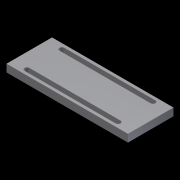
# Autodesk Inventor part: JointA3
Saved by Autodesk Inventor 2011 (Build 150239000, 239)
## iProperties
Created: 2012-10-15
Part Number: JointA3
Document SubType Name: Modeling
Designer: JohnHenry
Density: 1 g/cm^3
Author: JohnHenry
Autodesk Inventor part; units mm, degrees
ref_plane "YZ Plane" through (0, 0, 0) normal (1, 0, 0) x (0, 1, 0)
ref_plane "XZ Plane" through (0, 0, 0) normal (0, 1, 0) x (-1, 0, 0)
ref_plane "XY Plane" through (0, 0, 0) normal (0, 0, 1) x (1, 0, 0)
sketch "スケッチ1" plane through (0, 0, 0) normal (0, 0, 1) x (1, 0, 0)
  line L0 (-40, 15) -> (40, 15)
  line L1 (40, 15) -> (40, -15)
  line L2 (40, -15) -> (-40, -15)
  line L3 (-40, -15) -> (-40, 15)
  point P0 (0, 0)
  dimension "d0" = 80
  dimension "d1" = 40
  dimension "d2" = 30
  dimension "d3" = 15
  constraints: 8 end point, 2 parallel, 1 horizontal, 1 perpendicular
  measures "d0" distance of L0.start L0.end
  measures "d1" distance from line of L3 point (0, 0)
  measures "d2" distance of L0.end L1.end
  measures "d3" distance from line of point (0, 0) L2
extrude "押し出し1" add sketch "スケッチ1" along normal blind 5
sketch "スケッチ2" plane through (0, 0, 5) normal (0, 0, 1) x (1, 0, 0)
  line L0 (40, 15) -> (40, -15) projected
  line L1 (-40, 15) -> (40, 15) projected
  line L2 (-40, -15) -> (-40, 15) projected
  line L3 (40, -15) -> (-40, -15) projected
  line L4 (-30, 13.1) -> (30, 13.1)
  line L5 (30, 13.1) -> (30, 9.9)
  line L6 (30, 9.9) -> (-30, 9.9)
  line L7 (-30, 9.9) -> (-30, 13.1)
  line L8 (-30, -9.9) -> (30, -9.9)
  line L9 (30, -9.9) -> (30, -13.1)
  line L10 (30, -13.1) -> (-30, -13.1)
  line L11 (-30, -13.1) -> (-30, -9.9)
  circle A0 centre (-30, 11.5) radius 1.6
  circle A1 centre (30, 11.5) radius 1.6
  circle A2 centre (-30, -11.5) radius 1.6
  circle A3 centre (30, -11.5) radius 1.6
  point P0 (0, 0)
  dimension "d6" = 5.1
  dimension "d7" = 3.2
  dimension "d8" = 5.1
  dimension "d9" = 3.2
  dimension "d10" = 10
  dimension "d11" = 10
  dimension "d12" = 10
  dimension "d13" = 10
  constraints: 16 end point, 4 midpoint, 4 parallel, 4 vertical alignment, 2 horizontal, 2 perpendicular, 8 other
  measures "d6" distance between parallel lines of L6 L1
  measures "d7" distance of L6.end L4.start
  measures "d8" distance between parallel lines of L3 L8
  measures "d9" distance of L10.end L8.start
  measures "d10" distance between parallel lines of L2 L7
  measures "d11" distance between parallel lines of L2 L11
  measures "d12" distance between parallel lines of L0 L5
  measures "d13" distance between parallel lines of L9 L0
extrude "押し出し2" cut sketch "スケッチ2" against normal through all contours A0 L7 | L4 A1 L6 A0 | L7 A0 | A1 L5 | L5 A1 | A2 L11 | L8 A3 L10 A2 | L11 A2 | A3 L9 | L9 A3
equation "\"d1\" = 0.5 * d0"
equation "\"d3\" = 0.5 * d2"
equation "\"d8\" = d6"
equation "\"d9\" = d7"
equation "\"d11\" = d10"
equation "\"d12\" = d10"
equation "\"d13\" = d10"
